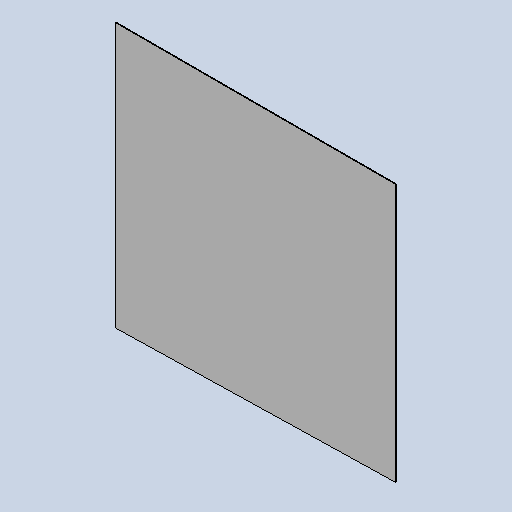
# Autodesk Inventor part: GBK 2111 shield 1
Saved by Autodesk Inventor 2026.2 (Build 302298010, 298A)
## iProperties
Created: 2026-04-17
Part Number: GBK 2111 shield 1
Material: Steel
Document SubType Name: Sheet Metal
Designer: pokla
Stock Number: 2111
Mass: 69243.3 g
Surface Area: 44341.6 cm^2
Volume: 8820.8 cm^3
Density: 7.85 g/cm^3
Sheet Metal Rule: Default_mm
Sheet Metal Width: 0,000 mm
Sheet Metal Length: 0,000 mm
Sheet Metal Area: 0,000 mm^2
Appearance: Default
Author: admin
Autodesk Inventor part; units mm, degrees
ref_plane "YZ Plane" through (0, 0, 0) normal (1, 0, 0) x (0, 1, 0)
ref_plane "XZ Plane" through (0, 0, 0) normal (0, 1, 0) x (-1, 0, 0)
ref_plane "XY Plane" through (0, 0, 0) normal (0, 0, 1) x (1, 0, 0)
sketch "Sketch1" plane through (0, 0, 0) normal (0, 0, 1) x (1, 0, 0)
  line L0 (740, -745) -> (-740, -745)
  line L1 (-740, -745) -> (-740, 745)
  line L2 (-740, 745) -> (740, 745)
  line L3 (740, 745) -> (740, -745)
  line L4 (740, -745) -> (-740, 745) construction
  line L5 (-740, -745) -> (740, 745) construction
  line L6 (-740, -652) -> (740, -618.4141)
  point P0 (0, 0)
  dimension "d0" = 1480
  dimension "d1" = 1490
  dimension "d3" = 1.3
  dimension "d4" = 93
  measures "d0" distance of L1.end L2.end
  measures "d1" distance of L0.end L1.end
  measures "d3" angle of L0 L6
  measures "d4" distance of L0.end L6.start
extrude "Plate1" add sketch "Sketch1" along normal blind 4 contours L6 L1 L2 L3
sketch "Sketch3" plane through (0, 0, 0) normal (0, 0, -1) x (-1, 0, 0)
  line L0 (562.4602, -535.2203) -> (562.4602, -892.9108) construction
  line L1 (562.4602, -892.9108) -> (533.3905, -892.9108) construction
  line L2 (533.3905, -892.9108) -> (533.3905, -535.2203) construction
  line L3 (533.3905, -535.2203) -> (562.4602, -535.2203) construction
  line L4 (710, -491.5) -> (770, -491.5) projected
  line L5 (710, -491.5) -> (710, -487.5) projected
  line L6 (669.8628, -495) -> (669.8628, -592) projected
  line L7 (669.8628, -592) -> (665.8638, -592) projected
  line L8 (710, 5.1667) -> (770, 5.1667) projected
  line L9 (710, 5.1667) -> (710, 9.1667) projected
  line L10 (710, 501.8333) -> (770, 501.8333) projected
  line L11 (710, 501.8333) -> (710, 505.8333) projected
  ellipse E0 centre (669.8628, 743) end of major axis (669.8628, 773) minor radius 0.6803 (669.8628, 713) -> (669.8628, 773) ccw projected
  line L12 (669.8628, 713) -> (665.8638, 713) projected
  ellipse E1 centre (169.7342, 743) end of major axis (169.7342, 773) minor radius 0.6803 (169.7342, 713) -> (169.7342, 773) ccw projected
  line L13 (169.7342, 713) -> (165.7352, 713) projected
  ellipse E2 centre (-330.3944, 743) end of major axis (-330.3944, 773) minor radius 0.6803 (-330.3944, 713) -> (-330.3944, 773) ccw projected
  line L14 (-330.3944, 713) -> (-334.3934, 713) projected
  line L15 (-738.6395, 501.8333) -> (-680, 501.8333) projected
  line L16 (-680, 501.8333) -> (-680, 505.8333) projected
  line L17 (-738.6395, 5.1667) -> (-680, 5.1667) projected
  line L18 (-680, 5.1667) -> (-680, 9.1667) projected
  line L19 (-738.6395, -491.5) -> (-680, -491.5) projected
  line L20 (-680, -491.5) -> (-680, -487.5) projected
  line L21 (-330.3944, -495) -> (-330.3944, -592) projected
  line L22 (-330.3944, -592) -> (-334.3934, -592) projected
  line L23 (169.7342, -495) -> (169.7342, -592) projected
  line L24 (169.7342, -592) -> (165.7352, -592) projected
  point P0 (0, 0)
  constraints: 5 other
mark "Mark2"
equation "\"d0\" = Лист_ширина"
equation "\"d1\" = 0.5 * Лист_длина"
equation "\"d2\" = Thickness"
equation "\"BendRadius\" = Thickness"
equation "\"BendReliefWidth\" = Thickness"
equation "\"BendReliefDepth\" = 0.5 * Thickness"
equation "\"CornerReliefSize\" = 4 * Thickness"
equation "\"MinimumRemnant\" = 2 * Thickness"
equation "\"TransitionRadius\" = BendRadius"
equation "\"JacobiRadiusSize\" = BendRadius"
equation "\"GapSize\" = Thickness"
equation "\"Лист_ширина\" = 1480"
equation "\"Лист_длина\" = 2980"
equation "\"Thickness\" = 4"
body "Solid1"
